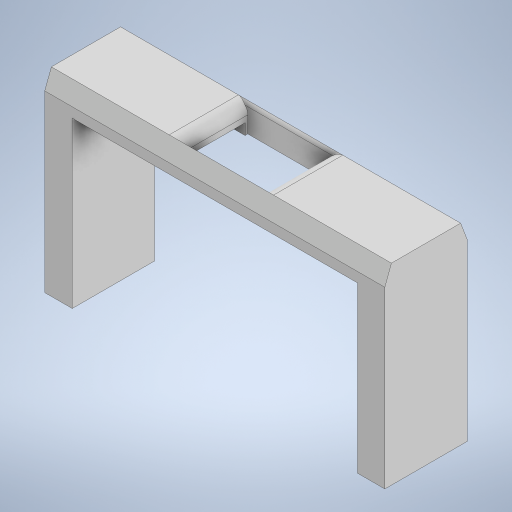
# Autodesk Inventor part: Landing dock
Saved by Autodesk Inventor 2023 (Build 270158000, 158)
## iProperties
Created: 2022-11-14
Part Number: Landing dock
Material: Generic
Document SubType Name: Modeling
Designer: cheng
Density: 1 g/cm^3
Appearance: Default
Author: cheng
Autodesk Inventor part; units mm, degrees
ref_plane "YZ Plane" through (0, 0, 0) normal (1, 0, 0) x (0, 1, 0)
ref_plane "XZ Plane" through (0, 0, 0) normal (0, 1, 0) x (-1, 0, 0)
ref_plane "XY Plane" through (0, 0, 0) normal (0, 0, 1) x (1, 0, 0)
sketch "Sketch1" plane through (0, 0, 0) normal (0, 1, 0) x (-1, 0, 0)
  line L0 (533.1208, -197.0984) -> (483.1208, -197.0984)
  line L1 (483.1208, -197.0984) -> (483.1208, -47.0984)
  line L2 (483.1208, -47.0984) -> (533.1208, -47.0984)
  line L3 (533.1208, -47.0984) -> (533.1208, -197.0984)
  line L4 (533.1208, -197.0984) -> (483.1208, -47.0984) construction
  line L5 (483.1208, -197.0984) -> (533.1208, -47.0984) construction
  line L6 (-35.8792, -197.0984) -> (-85.8792, -197.0984)
  line L7 (-85.8792, -197.0984) -> (-85.8792, -47.0984)
  line L8 (-85.8792, -47.0984) -> (-35.8792, -47.0984)
  line L9 (-35.8792, -47.0984) -> (-35.8792, -197.0984)
  line L10 (-35.8792, -197.0984) -> (-85.8792, -47.0984) construction
  line L11 (-85.8792, -197.0984) -> (-35.8792, -47.0984) construction
  point P0 (0, 0)
  point P1 (508.1208, -122.0984)
  point P2 (-60.8792, -122.0984)
  dimension "d1" = 150
  dimension "d2" = 150
  dimension "d3" = 619
  dimension "d4" = 50
  dimension "d5" = 50
  constraints: 24 end point, 4 midpoint, 4 parallel, 2 horizontal, 2 perpendicular, 1 point on line
  measures "d1" distance of L0.end L1.end
  measures "d2" distance of L8.end L6.start
  measures "d3" distance between parallel lines of L7 L3
  measures "d4" distance of L0.start L0.end
  measures "d5" distance of L6.start L6.end
extrude "Extrusion1" add sketch "Sketch1" along normal blind 300
sketch "Sketch2" plane through (0, 300, 0) normal (0, 1, 0) x (1, 0, 0)
  line L0 (-483.1208, 197.0984) -> (-533.1208, 197.0984) projected
  line L1 (35.8792, 47.0984) -> (85.8792, 47.0984) projected
  line L2 (-533.1208, 197.0984) -> (85.8792, 197.0984)
  line L3 (85.8792, 197.0984) -> (85.8792, 47.0984)
  line L4 (85.8792, 47.0984) -> (-533.1208, 47.0984)
  line L5 (-533.1208, 47.0984) -> (-533.1208, 197.0984)
  point P0 (0, 0)
  constraints: 8 end point, 2 parallel, 1 horizontal, 1 perpendicular
extrude "Extrusion2" add sketch "Sketch2" along normal blind 50
sketch "Sketch3" plane through (0, 350, 0) normal (0, 1, 0) x (1, 0, 0)
  line L0 (85.8792, 197.0984) -> (35.8792, 197.0984) construction
  line L1 (-533.1208, 47.0984) -> (-483.1208, 47.0984) construction
  line L2 (85.8792, 197.0984) -> (-533.1208, 47.0984) construction
  line L3 (85.8792, 47.0984) -> (85.8792, 197.0984) construction
  line L4 (-483.1208, 197.0984) -> (-533.1208, 197.0984) construction
  line L5 (85.8792, 47.0984) -> (-533.1208, 197.0984) construction
  line L6 (-148.6208, 62.0984) -> (-298.6208, 62.0984)
  line L7 (-298.6208, 62.0984) -> (-298.6208, 182.0984)
  line L8 (-298.6208, 182.0984) -> (-148.6208, 182.0984)
  line L9 (-148.6208, 182.0984) -> (-148.6208, 62.0984)
  line L10 (-148.6208, 62.0984) -> (-298.6208, 182.0984) construction
  line L11 (-298.6208, 62.0984) -> (-148.6208, 182.0984) construction
  point P0 (0, 0)
  point P1 (-223.6208, 122.0984)
  dimension "d12" = 120
  dimension "d13" = 150
  constraints: 16 end point, 3 midpoint, 2 parallel, 1 horizontal, 1 perpendicular
  measures "d12" distance of L8.end L6.start
  measures "d13" distance of L7.end L8.end
extrude "Extrusion3" cut sketch "Sketch3" against normal through all
sketch "Sketch4" plane through (85.8792, 0, -47.0984) normal (1, 0, 0) x (0, 0, -1)
  line L0 (0, 0) -> (0, 350) projected
  line L1 (150, 0) -> (150, 350) projected
  line L2 (0, 350) -> (150, 350)
  line L3 (150, 350) -> (150, 318)
  line L4 (150, 318) -> (0, 318)
  line L5 (0, 318) -> (0, 350)
  line L6 (150, 350) -> (0, 350) construction
  line L7 (150, 318) -> (0, 350) construction
  line L8 (0, 318) -> (150, 350) construction
  line L9 (12, 318) -> (12, 350)
  line L10 (75, 334) -> (75, 318) construction
  line L11 (75, 334) -> (75, 350) construction
  line L12 (15, 350) -> (135, 350) construction
  line L13 (0, 318) -> (12, 350)
  line L14 (138, 318) -> (138, 350)
  line L15 (150, 318) -> (138, 350)
  point P0 (-47.0984, 0)
  point P1 (0, 318)
  dimension "d14" = 32
  dimension "d15" = 12
  constraints: 24 end point, 3 midpoint, 3 point on line, 2 parallel, 2 perpendicular, 2 symmetric about line, 1 horizontal
  measures "d14" distance between parallel lines of L4 L2
  measures "d15" distance between parallel lines of L9 L0
extrude "Extrusion4" cut sketch "Sketch4" against normal through all contours L0 L2 L13 | L2 L1 L15
sketch "Sketch5" plane through (0, 300, 0) normal (0, -1, 0) x (1, 0, 0)
  line L0 (-298.6208, -182.0984) -> (-298.6208, -62.0984) projected
  line L1 (-148.6208, -182.0984) -> (-298.6208, -182.0984) projected
  line L2 (-298.6208, -62.0984) -> (-148.6208, -62.0984) projected
  line L3 (-148.6208, -62.0984) -> (-148.6208, -182.0984) projected
  line L4 (-298.6208, -62.0984) -> (-148.6208, -182.0984) construction
  line L5 (-298.6208, -182.0984) -> (-148.6208, -182.0984) construction
  line L6 (-148.6208, -62.0984) -> (-298.6208, -182.0984) construction
  line L7 (1.3792, -67.0984) -> (-448.6208, -67.0984)
  line L8 (-448.6208, -67.0984) -> (-448.6208, -177.0984)
  line L9 (-448.6208, -177.0984) -> (1.3792, -177.0984)
  line L10 (1.3792, -177.0984) -> (1.3792, -67.0984)
  line L11 (1.3792, -67.0984) -> (-448.6208, -177.0984) construction
  line L12 (-448.6208, -67.0984) -> (1.3792, -177.0984) construction
  point P0 (0, 0)
  point P1 (-223.6208, -122.0984)
  point P2 (-148.6208, -67.0984)
  point P3 (-148.6208, -177.0984)
  point P4 (-298.6208, -177.0984)
  point P5 (-298.6208, -67.0984)
  dimension "d18" = 450
  constraints: 16 end point, 3 midpoint, 2 parallel, 1 horizontal, 1 perpendicular
  measures "d18" distance of L7.start L7.end
extrude "Extrusion5" cut sketch "Sketch5" against normal blind 20 contours L9 L8 L7 L0 | L3 L7 L10 L9
fillet "Fillet1" radius 20 2 edges at (-148.6208, 350, -122.0984) (-298.6208, 350, -122.0984)
fillet "Fillet1" radius 10 2 edges at (-223.6208, 350, -62.0984) (-223.6208, 350, -182.0984)
body "Solid1"
